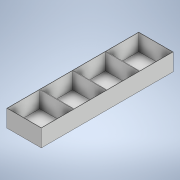
# Autodesk Inventor part: коробка ардуинкародина
Saved by Autodesk Inventor 2022.4 (Build 264492010, 492A)
## iProperties
Created: 2023-02-20
Part Number: коробка ардуинкародина
Material: Типовые
Document SubType Name: Modeling
Designer: artyo
Density: 1 g/cm^3
Appearance: По умолчанию
Author: artyo
Autodesk Inventor part; units mm, degrees
ref_plane "YZ Plane" through (0, 0, 0) normal (1, 0, 0) x (0, 1, 0)
ref_plane "XZ Plane" through (0, 0, 0) normal (0, 1, 0) x (-1, 0, 0)
ref_plane "XY Plane" through (0, 0, 0) normal (0, 0, 1) x (1, 0, 0)
sketch "Эскиз1" plane through (0, 0, 0) normal (0, 1, 0) x (-1, 0, 0)
  line L0 (-60, -230) -> (60, -230)
  line L1 (60, -230) -> (60, 230)
  line L2 (60, 230) -> (-60, 230)
  line L3 (-60, 230) -> (-60, -230)
  line L4 (-60, -230) -> (60, 230) construction
  line L5 (60, -230) -> (-60, 230) construction
  point P0 (0, 0)
  dimension "d0" = 120
  dimension "d1" = 460
  constraints: 12 end point, 2 midpoint, 2 parallel, 1 horizontal, 1 perpendicular
  measures "d0" distance of L2.end L1.end
  measures "d1" distance of L1.end L0.end
extrude "Выдавливание1" add sketch "Эскиз1" along normal blind 2
sketch "Эскиз3" plane through (0, 2, 0) normal (0, 1, 0) x (1, 0, 0)
  line L0 (59, -229) -> (-59, -229)
  line L1 (-59, -229) -> (-59, 229)
  line L2 (-59, 229) -> (59, 229)
  line L3 (59, 229) -> (59, -229)
  line L4 (59, -229) -> (-59, 229) construction
  line L5 (-59, -229) -> (59, 229) construction
  line L6 (59, -229) -> (-59, -229)
  line L7 (-59, -229) -> (-59, -116.5)
  line L8 (-59, -116.5) -> (59, -116.5)
  line L9 (59, -116.5) -> (59, -229)
  line L10 (-59, -116.5) -> (59, -116.5)
  line L11 (59, -116.5) -> (59, -114.5)
  line L12 (59, -114.5) -> (-59, -114.5)
  line L13 (-59, -114.5) -> (-59, -116.5)
  line L14 (59, -114.5) -> (-59, -114.5)
  line L15 (-59, -114.5) -> (-59, -2)
  line L16 (-59, -2) -> (59, -2)
  line L17 (59, -2) -> (59, -114.5)
  line L18 (59, -2) -> (-59, -2)
  line L19 (-59, -2) -> (-59, 0)
  line L20 (-59, 0) -> (59, 0)
  line L21 (59, 0) -> (59, -2)
  line L22 (-59, 0) -> (59, 0)
  line L23 (59, 0) -> (59, 112.5)
  line L24 (59, 112.5) -> (-59, 112.5)
  line L25 (-59, 112.5) -> (-59, 0)
  line L26 (-59, 112.5) -> (59, 112.5)
  line L27 (59, 112.5) -> (59, 114.5)
  line L28 (59, 114.5) -> (-59, 114.5)
  line L29 (-59, 114.5) -> (-59, 112.5)
  line L30 (-59, 114.5) -> (59, 114.5)
  line L31 (59, 114.5) -> (59, 229)
  line L32 (59, 229) -> (-59, 229)
  line L33 (-59, 229) -> (-59, 114.5)
  line L34 (-60, 230) -> (-60, -230) projected
  line L35 (60, -230) -> (60, 230) projected
  line L36 (-60, -230) -> (60, -230)
  line L37 (60, -230) -> (60, 230)
  line L38 (60, 230) -> (-60, 230)
  line L39 (-60, 230) -> (-60, -230)
  point P0 (0, 0)
  point P1 (59, -116.5)
  point P2 (59, 0)
  point P3 (-59, 112.5)
  dimension "d14" = 118
  dimension "d15" = 458
  dimension "d16" = 112.5
  dimension "d17" = 118
  dimension "d18" = 2
  dimension "d19" = 118
  dimension "d20" = 112.5
  dimension "d21" = 118
  dimension "d22" = 112.5
  dimension "d23" = 118
  dimension "d24" = 2
  constraints: 76 end point, 18 parallel, 9 horizontal, 9 perpendicular, 3 midpoint, 1 point on line
  measures "d14" distance of L1.end L2.end
  measures "d15" distance of L0.end L1.end
  measures "d16" distance of L6.end L7.end
  measures "d17" distance of L7.end L8.end
  measures "d18" distance of L11.end L10.end
  measures "d19" distance of L15.end L16.end
  measures "d20" distance of L14.end L15.end
  measures "d21" distance of L24.end L23.end
  measures "d22" distance of L23.end L22.end
  measures "d23" distance of L28.end L27.end
  measures "d24" distance of L27.end L26.end
extrude "Выдавливание3" add sketch "Эскиз3" along normal blind 58 contours L8 L1 L12 L3 | L16 L1 L20 L3 | L24 L1 L28 L3 | L38 L35 L36 L34
